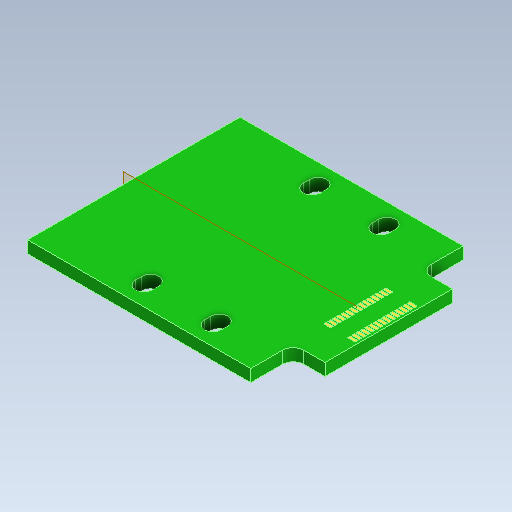
# Autodesk Inventor part: Extension PCB
Saved by Autodesk Inventor 2021 (Build 250183000, 183)
## iProperties
Created: 2020-04-17
Part Number: Extension PCB
Material: Generic
Document SubType Name: Modeling
Designer: jgray
Density: 1 g/cm^3
Appearance: Default
Author: jgray
Autodesk Inventor part; units mm, degrees
ref_plane "YZ Plane" through (0, 0, 0) normal (1, 0, 0) x (0, 1, 0)
ref_plane "XZ Plane" through (0, 0, 0) normal (0, 1, 0) x (-1, 0, 0)
ref_plane "XY Plane" through (0, 0, 0) normal (0, 0, 1) x (1, 0, 0)
sketch "Sketch1" plane through (0, 0, 0) normal (0, 1, 0) x (-1, 0, 0)
  line L0 (0, 0) -> (48, 0)
  line L1 (48, 0) -> (48, -40)
  line L2 (48, -40) -> (0, -40)
  line L3 (0, -40) -> (0, 0)
  dimension "d0" = 48
  dimension "d1" = 40
  constraints: 8 end point, 2 parallel, 1 horizontal, 1 perpendicular
  measures "d0" distance of L1.end L2.end
  measures "d1" distance of L0.end L1.end
extrude "Extrusion1" add sketch "Sketch1" along normal blind 2.3
sketch "Sketch2" plane through (0, 2.3, 0) normal (0, 1, 0) x (1, 0, 0)
  line L0 (-50.9993, 20) -> (5.4412, 20) construction
  line L1 (-50.9993, 4.2) -> (11.1887, 4.2) construction
  line L2 (-50.9993, 35.8) -> (7.0505, 35.8) construction
  line L3 (-48, 40) -> (-48, 0) construction
  line L4 (-29.7, 3.6) -> (-29.7, 4.8) construction
  line L5 (-28.1, 3.6) -> (-28.1, 4.8)
  line L6 (-31.3, 4.8) -> (-31.3, 3.6)
  arc A0 (-31.3, 3.6) -> (-28.1, 3.6) centre (-29.7, 3.6) ccw
  arc A1 (-28.1, 4.8) -> (-31.3, 4.8) centre (-29.7, 4.8) ccw
  line L7 (-33.7213, 4.2) -> (28.4668, 4.2) construction
  line L8 (-16.7, 3.6) -> (-16.7, 4.8) construction
  line L9 (-15.1, 3.6) -> (-15.1, 4.8)
  line L10 (-18.3, 4.8) -> (-18.3, 3.6)
  arc A2 (-18.3, 3.6) -> (-15.1, 3.6) centre (-16.7, 3.6) ccw
  arc A3 (-15.1, 4.8) -> (-18.3, 4.8) centre (-16.7, 4.8) ccw
  line L11 (0, 0) -> (0, 40) projected
  line L12 (-29.7, 35.2) -> (-29.7, 36.4) construction
  line L13 (-31.3, 35.2) -> (-31.3, 36.4)
  line L14 (-28.1, 36.4) -> (-28.1, 35.2)
  arc A4 (-31.3, 35.2) -> (-28.1, 35.2) centre (-29.7, 35.2) ccw
  arc A5 (-28.1, 36.4) -> (-31.3, 36.4) centre (-29.7, 36.4) ccw
  line L15 (-16.7, 35.2) -> (-16.7, 36.4) construction
  line L16 (-18.3, 35.2) -> (-18.3, 36.4)
  line L17 (-15.1, 36.4) -> (-15.1, 35.2)
  arc A6 (-18.3, 35.2) -> (-15.1, 35.2) centre (-16.7, 35.2) ccw
  arc A7 (-15.1, 36.4) -> (-18.3, 36.4) centre (-16.7, 36.4) ccw
  point P0 (-48, 20)
  point P1 (-29.7, 4.2)
  point P2 (-16.7, 4.2)
  point P3 (-29.7, 35.8)
  point P4 (-16.7, 35.8)
  dimension "d4" = 31.6
  dimension "d5" = 3.2
  dimension "d6" = 1.2
  dimension "d7" = 3.2
  dimension "d8" = 1.2
  dimension "d9" = 16.7
  dimension "d10" = 29.7
  constraints: 40 end point, 16 point on circle, 8 centre point, 8 tangent, 4 horizontal, 3 midpoint, 2 parallel, 2 point on line, 1 other
  measures "d4" distance between parallel lines of L2 L1
  measures "d5" diameter of A1
  measures "d6" distance of L4.end L4.start
  measures "d7" diameter of A3
  measures "d8" distance of L8.end L8.start
  measures "d9" distance from line of L11 point (-16.7, 4.2)
  measures "d10" distance from line of L11 point (-29.7, 4.2)
extrude "Extrusion2" cut sketch "Sketch2" against normal through all
sketch "Sketch3" plane through (0, 2.3, 0) normal (0, 1, 0) x (1, 0, 0)
  arc A0 (-31.3, 35.2) -> (-28.1, 35.2) centre (-29.7, 35.2) ccw construction
  line L0 (-31.3, 35.2) -> (-31.3, 36.4) construction
  arc A1 (-28.1, 36.4) -> (-31.3, 36.4) centre (-29.7, 36.4) ccw construction
  line L1 (-28.1, 36.4) -> (-28.1, 35.2) construction
  line L2 (-15.1, 4.8) -> (-15.1, 3.6) construction
  arc A2 (-18.3, 3.6) -> (-15.1, 3.6) centre (-16.7, 3.6) ccw construction
  line L3 (-18.3, 3.6) -> (-18.3, 4.8) construction
  arc A3 (-15.1, 4.8) -> (-18.3, 4.8) centre (-16.7, 4.8) ccw construction
  line L4 (-15.1, 36.4) -> (-15.1, 35.2) construction
  arc A4 (-18.3, 35.2) -> (-15.1, 35.2) centre (-16.7, 35.2) ccw construction
  line L5 (-18.3, 35.2) -> (-18.3, 36.4) construction
  arc A5 (-15.1, 36.4) -> (-18.3, 36.4) centre (-16.7, 36.4) ccw construction
  line L6 (-31.3, 3.6) -> (-31.3, 4.8) construction
  arc A6 (-28.1, 4.8) -> (-31.3, 4.8) centre (-29.7, 4.8) ccw construction
  line L7 (-28.1, 4.8) -> (-28.1, 3.6) construction
  arc A7 (-31.3, 3.6) -> (-28.1, 3.6) centre (-29.7, 3.6) ccw construction
  line L8 (0, 0) -> (0, 40) construction
  line L9 (0, 40) -> (-48, 40) construction
  line L10 (-48, 40) -> (-48, 0) construction
  line L11 (-48, 0) -> (0, 0) construction
  line L12 (-0.5, -4.3742) -> (-0.5, 50.5) construction
  line L13 (-1.9, -4.3742) -> (-1.9, 45.3415) construction
  line L14 (1.3314, 20) -> (-14.5, 20) construction
  line L15 (-1.9, 19.75) -> (-0.5, 19.75)
  line L16 (-0.5, 19.75) -> (-0.5, 20.25)
  line L17 (-0.5, 20.25) -> (-1.9, 20.25)
  line L18 (-1.9, 20.25) -> (-1.9, 19.75)
  line L19 (-6.4, 19.75) -> (-5.1, 19.75)
  line L20 (-5.1, 19.75) -> (-5.1, 20.25)
  line L21 (-5.1, 20.25) -> (-6.4, 20.25)
  line L22 (-6.4, 20.25) -> (-6.4, 19.75)
  line L23 (-6.4, 21.05) -> (-6.4, 20.55)
  line L24 (-5.1, 20.55) -> (-5.1, 21.05)
  line L25 (-5.1, 21.05) -> (-6.4, 21.05)
  line L26 (-6.4, 20.55) -> (-5.1, 20.55)
  line L27 (-1.9, 21.05) -> (-1.9, 20.55)
  line L28 (-0.5, 20.55) -> (-0.5, 21.05)
  line L29 (-1.9, 20.55) -> (-0.5, 20.55)
  line L30 (-0.5, 21.05) -> (-1.9, 21.05)
  line L31 (-6.4, 21.85) -> (-6.4, 21.35)
  line L32 (-5.1, 21.35) -> (-5.1, 21.85)
  line L33 (-5.1, 21.85) -> (-6.4, 21.85)
  line L34 (-6.4, 21.35) -> (-5.1, 21.35)
  line L35 (-1.9, 21.85) -> (-1.9, 21.35)
  line L36 (-0.5, 21.35) -> (-0.5, 21.85)
  line L37 (-1.9, 21.35) -> (-0.5, 21.35)
  line L38 (-0.5, 21.85) -> (-1.9, 21.85)
  line L39 (-6.4, 22.65) -> (-6.4, 22.15)
  line L40 (-5.1, 22.15) -> (-5.1, 22.65)
  line L41 (-5.1, 22.65) -> (-6.4, 22.65)
  line L42 (-6.4, 22.15) -> (-5.1, 22.15)
  line L43 (-1.9, 22.65) -> (-1.9, 22.15)
  line L44 (-0.5, 22.15) -> (-0.5, 22.65)
  line L45 (-1.9, 22.15) -> (-0.5, 22.15)
  line L46 (-0.5, 22.65) -> (-1.9, 22.65)
  line L47 (-6.4, 23.45) -> (-6.4, 22.95)
  line L48 (-5.1, 22.95) -> (-5.1, 23.45)
  line L49 (-5.1, 23.45) -> (-6.4, 23.45)
  line L50 (-6.4, 22.95) -> (-5.1, 22.95)
  line L51 (-1.9, 23.45) -> (-1.9, 22.95)
  line L52 (-0.5, 22.95) -> (-0.5, 23.45)
  line L53 (-1.9, 22.95) -> (-0.5, 22.95)
  line L54 (-0.5, 23.45) -> (-1.9, 23.45)
  line L55 (-6.4, 24.25) -> (-6.4, 23.75)
  line L56 (-5.1, 23.75) -> (-5.1, 24.25)
  line L57 (-5.1, 24.25) -> (-6.4, 24.25)
  line L58 (-6.4, 23.75) -> (-5.1, 23.75)
  line L59 (-1.9, 24.25) -> (-1.9, 23.75)
  line L60 (-0.5, 23.75) -> (-0.5, 24.25)
  line L61 (-1.9, 23.75) -> (-0.5, 23.75)
  line L62 (-0.5, 24.25) -> (-1.9, 24.25)
  line L63 (-6.4, 25.05) -> (-6.4, 24.55)
  line L64 (-5.1, 24.55) -> (-5.1, 25.05)
  line L65 (-5.1, 25.05) -> (-6.4, 25.05)
  line L66 (-6.4, 24.55) -> (-5.1, 24.55)
  line L67 (-1.9, 25.05) -> (-1.9, 24.55)
  line L68 (-0.5, 24.55) -> (-0.5, 25.05)
  line L69 (-1.9, 24.55) -> (-0.5, 24.55)
  line L70 (-0.5, 25.05) -> (-1.9, 25.05)
  line L71 (-6.4, 25.85) -> (-6.4, 25.35)
  line L72 (-5.1, 25.35) -> (-5.1, 25.85)
  line L73 (-5.1, 25.85) -> (-6.4, 25.85)
  line L74 (-6.4, 25.35) -> (-5.1, 25.35)
  line L75 (-1.9, 25.85) -> (-1.9, 25.35)
  line L76 (-0.5, 25.35) -> (-0.5, 25.85)
  line L77 (-1.9, 25.35) -> (-0.5, 25.35)
  line L78 (-0.5, 25.85) -> (-1.9, 25.85)
  line L79 (-0.5, 19.45) -> (-1.9, 19.45)
  line L80 (-1.9, 18.95) -> (-0.5, 18.95)
  line L81 (-1.9, 19.45) -> (-1.9, 18.95)
  line L82 (-0.5, 18.95) -> (-0.5, 19.45)
  line L83 (-5.1, 19.45) -> (-6.4, 19.45)
  line L84 (-6.4, 18.95) -> (-5.1, 18.95)
  line L85 (-5.1, 18.95) -> (-5.1, 19.45)
  line L86 (-6.4, 19.45) -> (-6.4, 18.95)
  line L87 (-0.5, 18.65) -> (-1.9, 18.65)
  line L88 (-1.9, 18.15) -> (-0.5, 18.15)
  line L89 (-1.9, 18.65) -> (-1.9, 18.15)
  line L90 (-0.5, 18.15) -> (-0.5, 18.65)
  line L91 (-5.1, 18.65) -> (-6.4, 18.65)
  line L92 (-6.4, 18.15) -> (-5.1, 18.15)
  line L93 (-5.1, 18.15) -> (-5.1, 18.65)
  line L94 (-6.4, 18.65) -> (-6.4, 18.15)
  line L95 (-0.5, 17.85) -> (-1.9, 17.85)
  line L96 (-1.9, 17.35) -> (-0.5, 17.35)
  line L97 (-1.9, 17.85) -> (-1.9, 17.35)
  line L98 (-0.5, 17.35) -> (-0.5, 17.85)
  line L99 (-5.1, 17.85) -> (-6.4, 17.85)
  line L100 (-6.4, 17.35) -> (-5.1, 17.35)
  line L101 (-5.1, 17.35) -> (-5.1, 17.85)
  line L102 (-6.4, 17.85) -> (-6.4, 17.35)
  line L103 (-0.5, 17.05) -> (-1.9, 17.05)
  line L104 (-1.9, 16.55) -> (-0.5, 16.55)
  line L105 (-1.9, 17.05) -> (-1.9, 16.55)
  line L106 (-0.5, 16.55) -> (-0.5, 17.05)
  line L107 (-5.1, 17.05) -> (-6.4, 17.05)
  line L108 (-6.4, 16.55) -> (-5.1, 16.55)
  line L109 (-5.1, 16.55) -> (-5.1, 17.05)
  line L110 (-6.4, 17.05) -> (-6.4, 16.55)
  line L111 (-0.5, 16.25) -> (-1.9, 16.25)
  line L112 (-1.9, 15.75) -> (-0.5, 15.75)
  line L113 (-1.9, 16.25) -> (-1.9, 15.75)
  line L114 (-0.5, 15.75) -> (-0.5, 16.25)
  line L115 (-5.1, 16.25) -> (-6.4, 16.25)
  line L116 (-6.4, 15.75) -> (-5.1, 15.75)
  line L117 (-5.1, 15.75) -> (-5.1, 16.25)
  line L118 (-6.4, 16.25) -> (-6.4, 15.75)
  line L119 (-0.5, 15.45) -> (-1.9, 15.45)
  line L120 (-1.9, 14.95) -> (-0.5, 14.95)
  line L121 (-1.9, 15.45) -> (-1.9, 14.95)
  line L122 (-0.5, 14.95) -> (-0.5, 15.45)
  line L123 (-5.1, 15.45) -> (-6.4, 15.45)
  line L124 (-6.4, 14.95) -> (-5.1, 14.95)
  line L125 (-5.1, 14.95) -> (-5.1, 15.45)
  line L126 (-6.4, 15.45) -> (-6.4, 14.95)
  line L127 (-0.5, 14.65) -> (-1.9, 14.65)
  line L128 (-1.9, 14.15) -> (-0.5, 14.15)
  line L129 (-1.9, 14.65) -> (-1.9, 14.15)
  line L130 (-0.5, 14.15) -> (-0.5, 14.65)
  line L131 (-5.1, 14.65) -> (-6.4, 14.65)
  line L132 (-6.4, 14.15) -> (-5.1, 14.15)
  line L133 (-5.1, 14.15) -> (-5.1, 14.65)
  line L134 (-6.4, 14.65) -> (-6.4, 14.15)
  point P0 (0, 20)
  point P1 (-1.9, 20)
  point P2 (-6.4, 20)
  point P3 (-6.4, 20.8)
  point P4 (-1.9, 20.8)
  point P5 (0, 20.8)
  point P6 (-6.4, 21.6)
  point P7 (-1.9, 21.6)
  point P8 (0, 21.6)
  point P9 (-6.4, 22.4)
  point P10 (-1.9, 22.4)
  point P11 (0, 22.4)
  point P12 (-6.4, 23.2)
  point P13 (-1.9, 23.2)
  point P14 (0, 23.2)
  point P15 (-6.4, 24)
  point P16 (-1.9, 24)
  point P17 (0, 24)
  point P18 (-6.4, 24.8)
  point P19 (-1.9, 24.8)
  point P20 (0, 24.8)
  point P21 (-6.4, 25.6)
  point P22 (-1.9, 25.6)
  point P23 (0, 25.6)
  point P24 (-1.9, 19.2)
  point P25 (-6.4, 19.2)
  point P26 (-1.9, 18.4)
  point P27 (-6.4, 18.4)
  point P28 (-1.9, 17.6)
  point P29 (-6.4, 17.6)
  point P30 (-1.9, 16.8)
  point P31 (-6.4, 16.8)
  point P32 (-1.9, 16)
  point P33 (-6.4, 16)
  point P34 (-1.9, 15.2)
  point P35 (-6.4, 15.2)
  point P36 (-1.9, 14.4)
  point P37 (-6.4, 14.4)
  dimension "d13" = 0.5
  dimension "d14" = 1.4
  dimension "d15" = 0.5
  dimension "d16" = 1.3
  dimension "d17" = 0.5
  dimension "d18" = 6.4
  dimension "d21" = 0.8
  dimension "d28" = 0.8
  constraints: 246 end point, 5 point on line, 4 parallel, 4 vertical, 3 horizontal, 3 midpoint, 2 perpendicular, 259 other
  measures "d13" distance between parallel lines of L8 L12
  measures "d14" distance between parallel lines of L13 L12
  measures "d15" distance between parallel lines of L17 L15
  measures "d16" distance of L21.end L20.end
  measures "d17" distance of L20.end L19.end
  measures "d18" distance between parallel lines of L8 L22
  measures "d21" distance of point (-6.4, 20) point (-6.4, 20.8)
  measures "d28" distance of L16.end L79.start
extrude "Extrusion3" add sketch "Sketch3" along normal blind 0.01
ref_plane "Work Plane1" through (-48, 2.3, -20) normal (0, 0, 1) x (1, 0, 0)
sketch "Sketch4" plane through (0, 2.3, 0) normal (0, 1, 0) x (1, 0, 0)
  line L0 (0, 0) -> (0, 40) projected
  line L1 (0, 40) -> (-6, 40)
  line L2 (-6, 40) -> (-6, 34)
  line L3 (-4, 32) -> (0, 32)
  line L4 (0, 32) -> (0, 40)
  arc A0 (-6, 34) -> (-4, 32) centre (-4, 34) ccw
  line L5 (4.4733, 20) -> (-53.814, 20) construction
  line L6 (0, 0) -> (-6, 0)
  line L7 (-6, 0) -> (-6, 6)
  line L8 (-4, 8) -> (0, 8)
  line L9 (0, 8) -> (0, 0)
  arc A1 (-4, 8) -> (-6, 6) centre (-4, 6) ccw
  point P0 (-6, 32)
  point P1 (0, 20)
  point P2 (-6, 8)
  dimension "d35" = 6
  dimension "d36" = 8
  dimension "d37" = 2
  constraints: 18 end point, 6 symmetric about line, 5 point on line, 4 point on circle, 2 centre point, 2 horizontal, 2 parallel, 2 tangent, 1 midpoint, 1 perpendicular, 1 other
  measures "d35" distance of L3.end point (-6, 32)
  measures "d36" distance of point (-6, 32) L1.end
  measures "d37" radius of A0
extrude "Extrusion4" cut sketch "Sketch4" against normal through all
body "Solid1"
